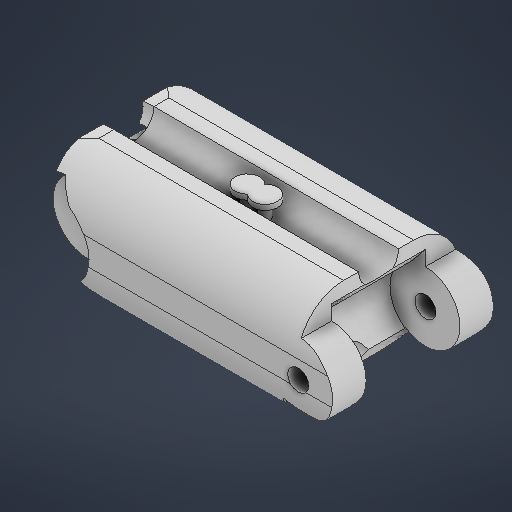
# Autodesk Inventor part: falange2_dedoGordo
Saved by Autodesk Inventor 2026.1 (Build 301233020, 233B)
## iProperties
Created: 2026-01-14
Part Number: falange2_dedoGordo
Material: Generic
Document SubType Name: Modeling
Designer: user
Density: 1 g/cm^3
Appearance: Default
Author: user
Autodesk Inventor part; units mm, degrees
ref_plane "YZ Plane" through (0, 0, 0) normal (1, 0, 0) x (0, 1, 0)
ref_plane "XY Plane" through (0, 0, 0) normal (0, 0, 1) x (1, 0, 0)
sketch "Sketch1" plane through (0, 0, 0) normal (0, 0, 1) x (1, 0, 0)
  line L0 (5.2681, -7.5236) -> (29.7319, -7.5236)
  circle A0 centre (0, 0) radius 1.5
  line L1 (0, 5) -> (0, 9.2)
  circle A1 centre (35, 0) radius 1.5
  arc A2 (32.1751, -4.0343) -> (35, 4.925) centre (35, 0) ccw
  line L2 (35, 4.925) -> (35, 9.075)
  line L3 (35, 9.075) -> (0, 9.2)
  arc A3 (0, 5) -> (2.8679, -4.0958) centre (0, 0) ccw
  line L4 (2.8679, -4.0958) -> (5.2681, -7.5236)
  line L5 (32.1751, -4.0343) -> (29.7319, -7.5236)
  dimension "d13" = 3
  dimension "d36" = 3
  dimension "d37" = 9.85
  dimension "d65" = 0
  dimension "d66" = 35
  dimension "d67" = 4.15
  dimension "d73" = 10
  dimension "d112" = 4.2
  dimension "d144" = 55
  dimension "d151" = 55
  dimension "d152" = 2.8249
  dimension "d153" = 2.8679
  constraints: 12 end point, 4 centre point, 4 point on circle, 3 coincident, 2 vertical, 1 parallel
  measures "d13" diameter of A0
  measures "d36" diameter of A1
  measures "d37" diameter of A2
  measures "d65" vertical distance of point (0, 0) A1.centre
  measures "d66" distance of A1.centre point (0, 0)
  measures "d67" distance of L2.start L2.end
  measures "d73" diameter of A3
  measures "d112" distance of L1.start L1.end
  measures "d144" angle of L0 L4
  measures "d151" angle of L0 L5
  measures "d152" horizontal distance of L5.start A2.centre
  measures "d153" horizontal distance of point (0, 0) L4.start
extrude "Extrusion1" add sketch "Sketch1" along normal mid plane 23
sketch "Sketch4" plane through (0, 9.2, -11.5) normal (-1, 0, 0) x (0, 0, 1)
  circle A0 centre (11.5, -13.8108) radius 1.5
  point P0 (11.5, -9.2)
  dimension "d23" = 3
  constraints: 1 centre point
  measures "d23" diameter of A0
extrude "Extrusion4" cut sketch "Sketch4" against normal through all
sketch "Sketch7" plane through (0, 0, 0) normal (0, 0, 1) x (1, 0, 0)
  circle A0 centre (35, 0) radius 5.075
  circle A1 centre (35, 0) radius 1.5 projected
  point P0 (0, 0)
  dimension "d116" = 10.15
  dimension "d154" = 0
  constraints: 1 centre point, 1 coincident
  measures "d116" diameter of A0
  measures "d154" distance of A1.centre point (35, 0)
extrude "Extrusion6" cut sketch "Sketch7" along normal mid plane 13.41 contours A0 | A1
sketch "Sketch12" plane through (0, 0, 11.5) normal (0, 0, 1) x (1, 0, 0)
  circle A0 centre (0, 0) radius 1.5 projected
  circle A1 centre (0, 0) radius 5.075
  dimension "d74" = 10.15
  constraints: 1 centre point, 1 coincident
  measures "d74" diameter of A1
extrude "Extrusion10" cut sketch "Sketch12" against normal blind 4.945
sketch "Sketch13" plane through (0, 0, -11.5) normal (0, 0, -1) x (-1, 0, 0)
  circle A0 centre (0, 0) radius 5.075
  dimension "d77" = 10.15
  constraints: 1 centre point
  measures "d77" diameter of A0
extrude "Extrusion11" cut sketch "Sketch13" against normal blind 4.945
sketch "Sketch14" plane through (0, 0, 0) normal (0, 0, 1) x (1, 0, 0)
  circle A0 centre (0, 0) radius 5
  dimension "d80" = 10
  constraints: 1 centre point, 1 coincident
  measures "d80" diameter of A0
extrude "Extrusion12" cut sketch "Sketch14" along normal mid plane 3.825
sketch "Sketch16" plane through (0, 0, 0) normal (0, 0, 1) x (1, 0, 0)
  circle A0 centre (0, 0) radius 1.5 projected
  line L0 (-1.9036, 2.4472) -> (1.1675, 2.8722)
  line L1 (1.1675, 2.8722) -> (3.0711, 0.425)
  line L2 (3.0711, 0.425) -> (1.9036, -2.4472)
  line L3 (1.9036, -2.4472) -> (-1.1675, -2.8722)
  line L4 (-1.1675, -2.8722) -> (-3.0711, -0.425)
  line L5 (-3.0711, -0.425) -> (-1.9036, 2.4472)
  dimension "d83" = 5.37
  constraints: 12 end point, 1 coincident, 13 other
  measures "d83" distance between parallel lines of L3 L0
extrude "Extrusion13" cut sketch "Sketch16" along normal mid plane 8.085 contours A0 | L0 L1 L2 L3 L4 L5
ref_plane "Work Plane1" through (0, 9.2, -11.5) normal (0, 1, 0) x (-1, 0, 0)
sketch "Sketch27" plane through (35, 4.925, -11.5) normal (1, 0, 0) x (0, 0, -1)
  line L0 (0, 4.15) -> (-23, 4.15) projected
  circle A0 centre (-11.5, 4.15) radius 2.8604
  point P0 (-11.5, -4.925)
  dimension "d117" = 5.7208
  constraints: 1 centre point, 1 midpoint
  measures "d117" diameter of A0
sketch "Sketch28" plane through (0, 9.2, 11.5) normal (0.0035714, 0.9999936, 0) x (0.9999936, -0.0035714, 0)
  line L0 (35.0002, 23) -> (35.0002, 0) projected
  line L1 (35.0002, 11.5) -> (0, 11.5)
  line L2 (0, 23) -> (0, 0) projected
  point P0 (0.0329, 11.5)
  constraints: 2 end point, 2 midpoint, 1 horizontal
sweep "Sweep1" cut profiles "Sketch27" path "Sketch28" path curves L1
ref_plane "Work Plane2" through (34.9898, 6.2146, 0) normal (0.0035714, 0.9999936, 0) x (0.9999936, -0.0035714, 0)
sketch "Sketch30" plane through (34.9898, 6.2146, 0) normal (0.0035714, 0.9999936, 0) x (0.9999936, -0.0035714, 0)
  line L0 (0.0143, -6.705) -> (0.0143, 6.705) projected
  line L1 (0.0143, 0) -> (-16.2257, 0)
  circle A0 centre (-16.2257, 0) radius 0.7321
  point P0 (-34.9674, 0)
  dimension "d122" = 16.24
  dimension "d123" = 1.4642
  constraints: 2 end point, 1 centre point, 1 coincident, 1 horizontal, 1 midpoint
  measures "d122" distance of L1.start L1.end
  measures "d123" diameter of A0
extrude "Extrusion19" add sketch "Sketch30" along normal blind 2.1075
sketch "Sketch31" plane through (18.7717, 8.3801, 0) normal (0.0035714, 0.9999936, 0) x (0.9999936, -0.0035714, 0)
  circle A0 centre (0, 0) radius 0.7321 projected
  circle A1 centre (0, 0) radius 1.774
  point P0 (-18.7417, 0)
  point P1 (-0.7321, 1.6159)
  point P2 (-0.7321, -1.6159)
  dimension "d126" = 3.548
  constraints: 2 point on circle, 1 centre point, 1 coincident
  measures "d126" diameter of A1
extrude "Extrusion20" add sketch "Sketch31" along normal up to surface (0.7529 mm away) contours A0 | A1
sketch "Sketch34" plane through (34.9898, 6.2146, 0) normal (0.0035714, 0.9999936, 0) x (0.9999936, -0.0035714, 0)
  ellipse E0 centre (0, 0) end of major axis (0, 2.8604) minor radius 0.0102 (0, -2.8604) -> (0, 2.8604) ccw projected
  ellipse E1 centre (-35.0002, 0) end of major axis (-35.0002, 2.8604) minor radius 0.0102 (-35.0002, -2.8604) -> (-35.0002, 2.8604) ccw projected
  line L0 (-35.0002, 0) -> (-18.7602, 0)
  circle A0 centre (-18.7602, 0) radius 0.7321
  point P0 (-34.9674, 0)
  dimension "d130" = 16.24
  dimension "d131" = 1.4642
  constraints: 2 end point, 1 centre point, 1 coincident, 1 horizontal, 2 other
  measures "d130" distance of L0.start L0.end
  measures "d131" diameter of A0
extrude "Extrusion21" add sketch "Sketch34" along normal blind 2.1075
sketch "Sketch35" plane through (16.2372, 8.3891, 0) normal (0.0035714, 0.9999936, 0) x (0.9999936, -0.0035714, 0)
  circle A0 centre (0, 0) radius 0.7321 projected
  circle A1 centre (0, 0) radius 1.774
  point P0 (-16.2071, 0)
  point P1 (0.7321, 0)
  point P2 (0.7321, 0)
  point P3 (-0.7321, 1.6159)
  point P4 (0.7321, -1.6159)
  point P5 (0.7321, 1.6159)
  dimension "d134" = 3.548
  constraints: 3 point on circle, 1 centre point, 1 coincident
  measures "d134" diameter of A1
extrude "Extrusion22" add sketch "Sketch35" along normal up to surface (0.7529 mm away) contours A0 | A1
chamfer "Chamfer1" distance 2 angle 45 1 edges at (35, 5.075, 0)
chamfer "Chamfer2" distance 2 angle 45 2 edges at (0, 5.075, -9.0275) (0, 5.075, 9.0275)
sketch "Sketch36" plane through (0, 5, -6.555) normal (-1, 0, 0) x (0, 0, 1)
  arc A0 (3.6946, 4.2) -> (9.4154, 4.2) centre (6.555, 4.2) ccw projected
  line L0 (18.055, 2.075) -> (13.11, 2.075) projected
  line L1 (9.4154, 4.2) -> (18.055, 4.2)
  line L2 (18.055, 4.2) -> (18.055, 2.075)
  line L3 (18.055, 2.075) -> (8.4697, 2.075)
  arc A1 (8.4697, 2.075) -> (9.4154, 4.2) centre (6.555, 4.2) ccw
  arc A2 (6.555, 1.3396) -> (9.4154, 4.2) centre (6.555, 4.2) ccw
  line L4 (6.555, 5.0268) -> (6.555, -0.0494)
  line L5 (-4.945, 2.075) -> (0, 2.075)
  line L6 (3.6946, 4.2) -> (-4.945, 4.2)
  line L7 (-4.945, 4.2) -> (-4.945, 2.075)
  line L8 (-4.945, 2.075) -> (4.6403, 2.075)
  arc A3 (3.6946, 4.2) -> (4.6403, 2.075) centre (6.555, 4.2) ccw
  line L9 (0, -10) -> (0, 0) projected
  line L10 (3.9417, -5) -> (10.0382, -5)
  point P0 (6.555, -5)
  point P1 (8.4697, 2.075)
  point P2 (13.11, 2.075)
  point P3 (0, 2.075)
  point P4 (4.6403, 2.075)
  constraints: 18 end point, 7 point on circle, 4 symmetric about line, 3 centre point, 2 coincident, 2 concentric, 2 horizontal, 1 parallel, 1 perpendicular, 1 vertical, 1 other
revolve "Revolution1" add sketch "Sketch36" angle 10 about axis through (0, 0, -2.6133) along (0, 0, 1)
fillet "Fillet1" radius 6.5 4 edges at (17.5, 9.1375, -11.5) (17.5, 9.1375, 11.5) (17.5, -7.5236, -11.5) (17.5, -7.5236, 11.5)
equation "\"d13\" = diametroDentroUnion"
equation "\"d36\" = diametroDentroUnion"
equation "\"d73\" = diametroFueraUnion"
equation "\"d80\" = diametroFueraUnion"
equation "\"d16\" = 135deg"
equation "\"d26\" = 135deg"
equation "\"d27\" = 135deg"
equation "\"d30\" = 135deg"
equation "\"d34\" = 23"
equation "\"d35\" = 0"
equation "\"d40\" = 135deg"
equation "\"d41\" = 10.639"
equation "\"d42\" = 11.8875"
equation "\"d43\" = 0"
equation "\"diametroDentroUnion\" = 3"
equation "\"diametroFueraUnion\" = 10"
equation "\"d45\" = 15"
equation "\"d39\" = diametroDentroUnion"
equation "\"tolerancia\" = 0.15"
body "Solid1"
